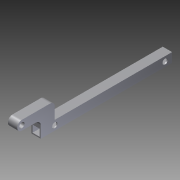
# Autodesk Inventor part: Arm
Saved by Autodesk Inventor 2012 (Build 160160000, 160)
## iProperties
Created: 2011-09-11
Part Number: Arm
Material: Default
Document SubType Name: Modeling
Designer: Ian Walters
Density: 1 g/cm^3
Author: Ian Walters
Autodesk Inventor part; units mm, degrees
ref_plane "YZ Plane" through (0, 0, 0) normal (1, 0, 0) x (0, 1, 0)
ref_plane "XZ Plane" through (0, 0, 0) normal (0, 1, 0) x (-1, 0, 0)
ref_plane "XY Plane" through (0, 0, 0) normal (0, 0, 1) x (1, 0, 0)
sketch "Sketch1" plane through (0, 0, 0) normal (0, 0, 1) x (1, 0, 0)
  line L0 (-25.4, 25.4) -> (25.4, 25.4)
  line L1 (25.4, 25.4) -> (25.4, -25.4)
  line L2 (25.4, -25.4) -> (-25.4, -25.4)
  line L3 (-25.4, -25.4) -> (-25.4, 25.4)
  line L4 (19.05, 19.05) -> (-19.05, 19.05)
  line L5 (-19.05, 19.05) -> (-19.05, -19.05)
  line L6 (-19.05, -19.05) -> (19.05, -19.05)
  line L7 (19.05, -19.05) -> (19.05, 19.05)
  point P0 (0, 0)
  point P1 (0, 25.4)
  point P2 (-25.4, 0)
  dimension "d0" = 50.8
  dimension "d1" = 50.8
  dimension "d2" = 6.35
  constraints: 16 end point, 4 parallel, 2 midpoint, 2 perpendicular, 1 horizontal, 1 horizontal alignment, 1 vertical alignment, 3 other
  measures "d0" distance of L0.start L0.end
  measures "d1" distance of L2.end L0.start
  measures "d2" distance between parallel lines of L3 L5
extrude "Extrusion1" add sketch "Sketch1" along normal mid plane 711.2
sketch "Sketch2" plane through (25.4, -25.4, 355.6) normal (1, 0, 0) x (0, 0, -1)
  line L0 (711.2, 0) -> (711.2, 50.8) projected
  circle A0 centre (673.1, 25.4) radius 14.2875
  line L1 (0, 50.8) -> (0, 0) projected
  circle A1 centre (76.2, 25.4) radius 14.2875
  point P0 (355.6, 25.4)
  point P1 (711.2, 25.4)
  point P2 (0, 25.4)
  dimension "d5" = 28.575
  dimension "d6" = 38.1
  dimension "d18" = 76.2
  constraints: 2 centre point, 2 horizontal alignment, 2 midpoint, 1 equal radius
  measures "d5" diameter of A0
  measures "d6" distance from line of L0 A0.centre
  measures "d18" distance from line of L1 A1.centre
extrude "Extrusion2" cut sketch "Sketch2" against normal up to surface (50.8 mm away)
sketch "Sketch3" plane through (25.4, -25.4, 355.6) normal (1, 0, 0) x (0, 0, -1)
  line L0 (0, 0) -> (711.2, 0) projected
  line L1 (0, 50.8) -> (711.2, 50.8) projected
  arc A0 (-101.6, 139.7) -> (-101.6, 88.9) centre (-101.6, 114.3) ccw
  circle A1 centre (-101.6, 114.3) radius 14.2875
  line L2 (-101.6, 88.9) -> (-25.4, 88.9)
  line L3 (-101.6, 139.7) -> (50.8, 139.7)
  line L4 (0, 50.8) -> (0, 63.5)
  line L5 (76.2, 114.3) -> (76.2, 50.8)
  arc A2 (76.2, 114.3) -> (50.8, 139.7) centre (50.8, 114.3) ccw
  arc A3 (0, 63.5) -> (-25.4, 88.9) centre (-25.4, 63.5) ccw
  point P0 (355.6, 25.4)
  point P1 (0, 88.9)
  point P2 (76.2, 139.7)
  dimension "d9" = 28.575
  dimension "d10" = 25.4
  dimension "d11" = 101.6
  dimension "d12" = 76.2
  dimension "d13" = 38.1
  dimension "d14" = 25.4
  constraints: 8 end point, 6 point on circle, 6 tangent, 5 point on line, 4 centre point, 2 parallel, 2 perpendicular, 1 coincident, 1 equal radius
  measures "d9" diameter of A1
  measures "d10" radius of A0
  measures "d11" distance of L2.start point (0, 88.9)
  measures "d12" distance from line of point (76.2, 139.7) L4
  measures "d13" distance between parallel lines of L2 L1
  measures "d14" radius of A2
extrude "Extrusion3" add sketch "Sketch3" against normal up to surface (50.8 mm away)
body "Solid1"
